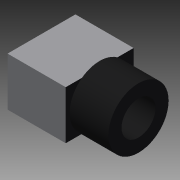
# Autodesk Inventor part: nanopc_t4_headphone
Saved by Autodesk Inventor 2013 SP2 (Build 170200200, 200)
## iProperties
Created: 2018-09-03
Part Number: nanopc_t4_headphone
Material: Generic
Document SubType Name: Modeling
Designer: alex
Density: 1 g/cm^3
Mass: 0.389415 g
Surface Area: 4.9487 cm^2
Volume: 0.389415 cm^3
Author: alex
Autodesk Inventor part; units mm, degrees
ref_plane "YZ Plane" through (0, 0, 0) normal (1, 0, 0) x (0, 1, 0)
ref_plane "XZ Plane" through (0, 0, 0) normal (0, 1, 0) x (-1, 0, 0)
ref_plane "Work Plane1" through (0, 0, 0) normal (0, 0, 1) x (1, 0, 0)
sketch "Sketch1" plane through (0, 0, 0) normal (0, 0, 1) x (1, 0, 0)
  line L0 (26.3787, 4.8051) -> (32.3787, 4.8051)
  line L1 (32.3787, 4.8051) -> (32.3787, -2.1949)
  line L2 (32.3787, -2.1949) -> (26.3787, -2.1949)
  line L3 (26.3787, -2.1949) -> (26.3787, 4.8051)
  point P0 (0, 0)
  dimension "d0" = 6
  dimension "d2" = 7
  constraints: 8 end point, 2 parallel, 1 horizontal, 1 perpendicular
  measures "d0" distance of L1.end L2.end
  measures "d2" distance of L0.end L1.end
extrude "Extrusion1" add sketch "Sketch1" along normal blind 5
sketch "Sketch2" plane through (32.3787, -2.1949, 0) normal (1, 0, 0) x (0, 0, -1)
  circle A0 centre (-2.5, 3.5) radius 3.1
  line L0 (0, 7) -> (-5, 7) projected
  line L1 (0, 0) -> (-5, 0) projected
  line L2 (-2.5, 3.5) -> (-2.5, 7)
  line L3 (-2.5, 3.5) -> (-2.5, 0)
  point P0 (0, 2.1949)
  dimension "d5" = 6.2
  constraints: 4 end point, 2 midpoint, 1 centre point, 1 collinear
  measures "d5" diameter of A0
extrude "Extrusion2" add sketch "Sketch2" along normal blind 4
sketch "Sketch3" plane through (36.3787, 1.3051, 2.5) normal (1, 0, 0) x (0, 0, -1)
  circle A0 centre (0, 0) radius 3.1 projected
  circle A1 centre (0, 0) radius 1.75
  point P0 (2.5, -1.3051)
  dimension "d9" = 3.5
  constraints: 1 centre point, 1 coincident
  measures "d9" diameter of A1
extrude "Extrusion3" cut sketch "Sketch3" against normal blind 7 contours A1
sketch "Sketch4" plane through (26.3787, -2.1949, 0) normal (-1, 0, 0) x (0, 0, 1)
  line L0 (0, 7) -> (5, 7) projected
  line L1 (5, 0) -> (2, 0)
  line L2 (2, 0) -> (2, 7)
  line L3 (2, 7) -> (5, 7)
  line L4 (5, 7) -> (5, 0)
  point P0 (0, 2.1949)
  dimension "d13" = 3
  constraints: 8 end point, 2 parallel, 1 horizontal, 1 perpendicular, 1 point on line
  measures "d13" distance between parallel lines of L4 L2
extrude "Extrusion4" add sketch "Sketch4" along normal blind 6
body "Solid1"
